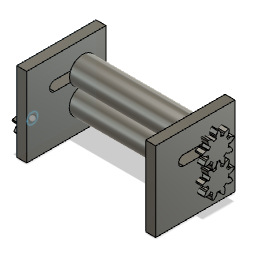
basic_parts (Autodesk Fusion 360 design; units mm, degrees)
Autodesk Fusion 360 part; units mm, degrees
sketch "biggear" plane through (0, 0, 0) normal (0, 1, 0) x (1, 0, 0)
  line L0 (141.1686, -145.633) -> (141.7294, -145.5695)
  line L1 (141.7294, -145.5695) -> (146.4127, -146.5108)
  line L2 (146.4127, -146.5108) -> (151.6977, -149.2435)
  line L3 (151.6977, -149.2435) -> (151.6977, -151.8334)
  line L4 (151.6977, -151.8334) -> (146.4127, -154.5661)
  line L5 (146.4127, -154.5661) -> (141.7294, -155.5074)
  line L6 (141.7294, -155.5074) -> (141.1687, -155.444)
  line L7 (141.1687, -155.444) -> (140.412, -159.9786)
  line L8 (140.412, -159.9786) -> (140.963, -160.1006)
  line L9 (140.963, -160.1006) -> (145.0868, -162.5116)
  line L10 (145.0868, -162.5116) -> (149.1982, -166.8123)
  line L11 (149.1982, -166.8123) -> (148.3573, -169.2618)
  line L12 (148.3573, -169.2618) -> (142.4713, -170.1304)
  line L13 (142.4713, -170.1304) -> (137.7361, -169.5001)
  line L14 (137.7361, -169.5001) -> (137.2263, -169.258)
  line L15 (137.2263, -169.258) -> (135.0383, -173.3012)
  line L16 (135.0383, -173.3012) -> (135.5198, -173.5955)
  line L17 (135.5198, -173.5955) -> (138.6373, -177.2149)
  line L18 (138.6373, -177.2149) -> (141.1295, -182.6175)
  line L19 (141.1295, -182.6175) -> (139.5388, -184.6613)
  line L20 (139.5388, -184.6613) -> (133.6897, -183.5717)
  line L21 (133.6897, -183.5717) -> (129.4158, -181.4379)
  line L22 (129.4158, -181.4379) -> (129.0122, -181.0435)
  line L23 (129.0122, -181.0435) -> (125.6299, -184.1571)
  line L24 (125.6299, -184.1571) -> (125.9897, -184.5919)
  line L25 (125.9897, -184.5919) -> (127.7632, -189.0274)
  line L26 (127.7632, -189.0274) -> (128.3661, -194.9465)
  line L27 (128.3661, -194.9465) -> (126.1979, -196.363)
  line L28 (126.1979, -196.363) -> (121.0195, -193.4332)
  line L29 (121.0195, -193.4332) -> (117.67, -190.0274)
  line L30 (117.67, -190.0274) -> (117.4164, -189.5232)
  line L31 (117.4164, -189.5232) -> (113.2064, -191.3699)
  line L32 (113.2064, -191.3699) -> (113.4055, -191.898)
  line L33 (113.4055, -191.898) -> (113.6427, -196.669)
  line L34 (113.6427, -196.669) -> (112.291, -202.4632)
  line L35 (112.291, -202.4632) -> (109.7804, -203.0989)
  line L36 (109.7804, -203.0989) -> (105.8339, -198.6465)
  line L37 (105.8339, -198.6465) -> (103.7717, -194.3376)
  line L38 (103.7717, -194.3376) -> (103.6955, -193.7784)
  line L39 (103.6955, -193.7784) -> (99.114, -194.158)
  line L40 (99.114, -194.158) -> (99.1309, -194.7221)
  line L41 (99.1309, -194.7221) -> (97.8061, -199.3117)
  line L42 (97.8061, -199.3117) -> (94.6462, -204.353)
  line L43 (94.6462, -204.353) -> (92.0652, -204.1391)
  line L44 (92.0652, -204.1391) -> (89.7783, -198.6465)
  line L45 (89.7783, -198.6465) -> (89.2269, -193.9015)
  line L46 (89.2269, -193.9015) -> (89.3365, -193.3478)
  line L47 (89.3365, -193.3478) -> (84.8799, -192.2193)
  line L48 (84.8799, -192.2193) -> (84.7127, -192.7583)
  line L49 (84.7127, -192.7583) -> (81.9694, -196.669)
  line L50 (81.9694, -196.669) -> (77.3439, -200.4112)
  line L51 (77.3439, -200.4112) -> (74.9722, -199.3708)
  line L52 (74.9722, -199.3708) -> (74.5926, -193.4332)
  line L53 (74.5926, -193.4332) -> (75.6118, -188.7663)
  line L54 (75.6118, -188.7663) -> (75.8952, -188.2782)
  line L55 (75.8952, -188.2782) -> (72.0465, -185.7638)
  line L56 (72.0465, -185.7638) -> (71.7134, -186.2193)
  line L57 (71.7134, -186.2193) -> (67.8489, -189.0274)
  line L58 (67.8489, -189.0274) -> (62.2589, -191.0649)
  line L59 (62.2589, -191.0649) -> (60.3535, -189.3108)
  line L60 (60.3535, -189.3108) -> (61.9225, -183.5716)
  line L61 (61.9225, -183.5716) -> (64.4018, -179.4885)
  line L62 (64.4018, -179.4885) -> (64.8283, -179.1189)
  line L63 (64.8283, -179.1189) -> (62.0046, -175.491)
  line L64 (62.0046, -175.491) -> (61.5416, -175.8137)
  line L65 (61.5416, -175.8137) -> (56.9748, -177.2149)
  line L66 (56.9748, -177.2149) -> (51.0261, -177.3269)
  line L67 (51.0261, -177.3269) -> (49.7935, -175.0492)
  line L68 (49.7935, -175.0492) -> (53.1409, -170.1304)
  line L69 (53.1409, -170.1304) -> (56.8117, -167.0736)
  line L70 (56.8117, -167.0736) -> (57.335, -166.8625)
  line L71 (57.335, -166.8625) -> (55.8423, -162.5143)
  line L72 (55.8423, -162.5143) -> (55.2996, -162.6692)
  line L73 (55.2996, -162.6692) -> (50.5253, -162.5116)
  line L74 (50.5253, -162.5116) -> (44.8626, -160.686)
  line L75 (44.8626, -160.686) -> (44.4363, -158.1315)
  line L76 (44.4363, -158.1315) -> (49.1995, -154.5661)
  line L77 (49.1995, -154.5661) -> (53.6639, -152.8668)
  line L78 (53.6639, -152.8668) -> (54.2275, -152.8371)
  line L79 (54.2275, -152.8371) -> (54.2275, -148.2398)
  line L80 (54.2275, -148.2398) -> (53.6639, -148.2101)
  line L81 (53.6639, -148.2101) -> (49.1995, -146.5108)
  line L82 (49.1995, -146.5108) -> (44.4363, -142.9454)
  line L83 (44.4363, -142.9454) -> (44.8626, -140.3909)
  line L84 (44.8626, -140.3909) -> (50.5253, -138.5654)
  line L85 (50.5253, -138.5654) -> (55.2996, -138.4077)
  line L86 (55.2996, -138.4077) -> (55.8423, -138.5626)
  line L87 (55.8423, -138.5626) -> (57.335, -134.2144)
  line L88 (57.335, -134.2144) -> (56.8117, -134.0033)
  line L89 (56.8117, -134.0033) -> (53.1409, -130.9465)
  line L90 (53.1409, -130.9465) -> (49.7934, -126.0277)
  line L91 (49.7934, -126.0277) -> (51.0261, -123.75)
  line L92 (51.0261, -123.75) -> (56.9748, -123.8621)
  line L93 (56.9748, -123.8621) -> (61.5416, -125.2632)
  line L94 (61.5416, -125.2632) -> (62.0046, -125.5859)
  line L95 (62.0046, -125.5859) -> (64.8283, -121.958)
  line L96 (64.8283, -121.958) -> (64.4018, -121.5884)
  line L97 (64.4018, -121.5884) -> (61.9225, -117.5053)
  line L98 (61.9225, -117.5053) -> (60.3535, -111.7661)
  line L99 (60.3535, -111.7661) -> (62.2589, -110.0121)
  line L100 (62.2589, -110.0121) -> (67.8489, -112.0496)
  line L101 (67.8489, -112.0496) -> (71.7134, -114.8576)
  line L102 (71.7134, -114.8576) -> (72.0465, -115.3132)
  line L103 (72.0465, -115.3132) -> (75.8952, -112.7987)
  line L104 (75.8952, -112.7987) -> (75.6118, -112.3106)
  line L105 (75.6118, -112.3106) -> (74.5926, -107.6437)
  line L106 (74.5926, -107.6437) -> (74.9722, -101.7061)
  line L107 (74.9722, -101.7061) -> (77.3439, -100.6657)
  line L108 (77.3439, -100.6657) -> (81.9694, -104.4079)
  line L109 (81.9694, -104.4079) -> (84.7127, -108.3186)
  line L110 (84.7127, -108.3186) -> (84.8799, -108.8576)
  line L111 (84.8799, -108.8576) -> (89.3364, -107.7291)
  line L112 (89.3364, -107.7291) -> (89.2269, -107.1755)
  line L113 (89.2269, -107.1755) -> (89.7783, -102.4305)
  line L114 (89.7783, -102.4305) -> (92.0652, -96.9378)
  line L115 (92.0652, -96.9378) -> (94.6462, -96.7239)
  line L116 (94.6462, -96.7239) -> (97.8061, -101.7653)
  line L117 (97.8061, -101.7653) -> (99.1309, -106.3548)
  line L118 (99.1309, -106.3548) -> (99.114, -106.9189)
  line L119 (99.114, -106.9189) -> (103.6955, -107.2985)
  line L120 (103.6955, -107.2985) -> (103.7717, -106.7393)
  line L121 (103.7717, -106.7393) -> (105.8339, -102.4305)
  line L122 (105.8339, -102.4305) -> (109.7804, -97.978)
  line L123 (109.7804, -97.978) -> (112.291, -98.6138)
  line L124 (112.291, -98.6138) -> (113.6427, -104.4079)
  line L125 (113.6427, -104.4079) -> (113.4055, -109.179)
  line L126 (113.4055, -109.179) -> (113.2064, -109.707)
  line L127 (113.2064, -109.707) -> (117.4164, -111.5537)
  line L128 (117.4164, -111.5537) -> (117.67, -111.0495)
  line L129 (117.67, -111.0495) -> (121.0195, -107.6437)
  line L130 (121.0195, -107.6437) -> (126.1979, -104.7139)
  line L131 (126.1979, -104.7139) -> (128.3661, -106.1304)
  line L132 (128.3661, -106.1304) -> (127.7632, -112.0496)
  line L133 (127.7632, -112.0496) -> (125.9897, -116.4851)
  line L134 (125.9897, -116.4851) -> (125.6299, -116.9198)
  line L135 (125.6299, -116.9198) -> (129.0122, -120.0335)
  line L136 (129.0122, -120.0335) -> (129.4158, -119.639)
  line L137 (129.4158, -119.639) -> (133.6897, -117.5053)
  line L138 (133.6897, -117.5053) -> (139.5388, -116.4156)
  line L139 (139.5388, -116.4156) -> (141.1295, -118.4594)
  line L140 (141.1295, -118.4594) -> (138.6373, -123.8621)
  line L141 (138.6373, -123.8621) -> (135.5198, -127.4814)
  line L142 (135.5198, -127.4814) -> (135.0383, -127.7757)
  line L143 (135.0383, -127.7757) -> (137.2263, -131.8189)
  line L144 (137.2263, -131.8189) -> (137.7361, -131.5768)
  line L145 (137.7361, -131.5768) -> (142.4713, -130.9465)
  line L146 (142.4713, -130.9465) -> (148.3573, -131.8151)
  line L147 (148.3573, -131.8151) -> (149.1982, -134.2646)
  line L148 (149.1982, -134.2646) -> (145.0868, -138.5653)
  line L149 (145.0868, -138.5653) -> (140.9629, -140.9763)
  line L150 (140.9629, -140.9763) -> (140.412, -141.0984)
  line L151 (140.412, -141.0984) -> (141.1686, -145.633)
sketch "smallgear" plane through (0, 0, 0) normal (0, 1, 0) x (-1, 0, 0)
  line L0 (42.6523, 16.1607) -> (47.1357, 13.5722)
  line L1 (64.2228, -1.5259) -> (58.7553, -4.5447)
  line L2 (43.751, 18.9194) -> (42.6523, 16.1607)
  line L3 (21.0334, -24.4753) -> (21.1528, -18.2309)
  line L4 (53.5978, -4.1821) -> (51.8271, -9.047)
  line L5 (54.4421, 9.3882) -> (51.8271, 7.9812)
  line L6 (56.9824, -19.4328) -> (50.8535, -18.2309)
  line L7 (58.2589, 16.8457) -> (56.011, 11.0187)
  line L8 (41.8813, -28.1514) -> (39.9256, -28.4962)
  line L9 (28.1014, 21.1769) -> (29.4347, 19.3487)
  line L10 (13.2511, 3.4789) -> (9.1458, 8.1857)
  line L11 (15.9953, -12.0844) -> (9.825, -11.1177)
  line L12 (22.7533, 24.4025) -> (28.1014, 21.1769)
  line L13 (21.1528, 17.1651) -> (21.0334, 23.4096)
  line L14 (56.011, 11.0187) -> (54.4421, 9.3882)
  line L15 (51.8271, 7.9812) -> (53.5978, 3.1164)
  line L16 (50.8535, 17.1651) -> (56.9824, 18.367)
  line L17 (35.4646, -18.4939) -> (30.3662, -17.5949)
  line L18 (48.9754, 15.9031) -> (50.8535, 17.1651)
  line L19 (22.7533, -25.4683) -> (21.0334, -24.4753)
  line L20 (41.8813, 27.0856) -> (43.9049, 21.1769)
  line L21 (58.7553, -4.5447) -> (56.5053, -4.7852)
  line L22 (56.5053, 3.7194) -> (58.7553, 3.4789)
  line L23 (9.1458, -9.2515) -> (13.2511, -4.5447)
  line L24 (51.8271, -9.047) -> (54.4421, -10.454)
  line L25 (9.1458, 8.1857) -> (9.825, 10.0519)
  line L26 (21.0334, 23.4096) -> (22.7533, 24.4025)
  line L27 (36.0032, 22.5702) -> (39.9256, 27.4305)
  line L28 (18.2215, 2.0556) -> (15.283, 2.4834)
  line L29 (9.825, 10.0519) -> (15.9953, 11.0187)
  line L30 (18.2215, -3.1214) -> (18.2215, 2.0556)
  line L31 (35.4646, 17.4281) -> (35.3756, 20.3962)
  line L32 (15.283, -3.5492) -> (18.2215, -3.1214)
  line L33 (13.2511, -4.5447) -> (15.283, -3.5492)
  line L34 (29.4347, 19.3487) -> (30.3662, 16.5291)
  line L35 (30.3662, 16.5291) -> (35.4646, 17.4281)
  line L36 (28.1014, -22.2427) -> (22.7533, -25.4683)
  line L37 (30.3662, -17.5949) -> (29.4347, -20.4144)
  line L38 (35.3756, -21.462) -> (35.4646, -18.4939)
  line L39 (43.9049, -22.2427) -> (41.8813, -28.1514)
  line L40 (39.9256, 27.4305) -> (41.8813, 27.0856)
  line L41 (56.011, -12.0844) -> (58.2589, -17.9115)
  line L42 (54.4421, -10.454) -> (56.011, -12.0844)
  line L43 (36.0032, -23.636) -> (35.3756, -21.462)
  line L44 (43.751, -19.9852) -> (43.9049, -22.2427)
  line L45 (56.5053, -4.7852) -> (53.5978, -4.1821)
  line L46 (47.1357, -14.638) -> (42.6523, -17.2265)
  line L47 (22.0695, 15.0964) -> (21.1528, 17.1651)
  line L48 (20.7178, 8.914) -> (24.0455, 12.8799)
  line L49 (15.283, 2.4834) -> (13.2511, 3.4789)
  line L50 (35.3756, 20.3962) -> (36.0032, 22.5702)
  line L51 (47.1357, 13.5722) -> (48.9754, 15.9031)
  line L52 (50.8535, -18.2309) -> (48.9754, -16.9689)
  line L53 (18.1918, -11.5409) -> (15.9953, -12.0844)
  line L54 (58.2589, -17.9115) -> (56.9824, -19.4328)
  line L55 (43.9049, 21.1769) -> (43.751, 18.9194)
  line L56 (22.0695, -16.1621) -> (24.0455, -13.9456)
  line L57 (9.825, -11.1177) -> (9.1458, -9.2515)
  line L58 (42.6523, -17.2265) -> (43.751, -19.9852)
  line L59 (64.2228, 0.4601) -> (64.2228, -1.5259)
  line L60 (39.9256, -28.4962) -> (36.0032, -23.636)
  line L61 (20.7178, -9.9798) -> (18.1918, -11.5409)
  line L62 (56.9824, 18.367) -> (58.2589, 16.8457)
  line L63 (58.7553, 3.4789) -> (64.2228, 0.4601)
  line L64 (29.4347, -20.4144) -> (28.1014, -22.2427)
  line L65 (24.0455, -13.9456) -> (20.7178, -9.9798)
  line L66 (15.9953, 11.0187) -> (18.1918, 10.4751)
  line L67 (24.0455, 12.8799) -> (22.0695, 15.0964)
  line L68 (48.9754, -16.9689) -> (47.1357, -14.638)
  line L69 (21.1528, -18.2309) -> (22.0695, -16.1621)
  line L70 (18.1918, 10.4751) -> (20.7178, 8.914)
  line L71 (53.5978, 3.1164) -> (56.5053, 3.7194)
scale "Scale1" [no effect]
scale "Scale2" [no effect]
extrude "Extrude3" add sketch "biggear" along normal blind 12.7 makes body 1
extrude "Extrude4" add sketch "smallgear" along normal blind 12.7 separate body makes body 2
cylinder "CylinderPrimitive1" add diameter 50.8 height 228.6 placed x (1, 0, 0) y (0, 0, -1) z (0, 1, 0) at (-75, 0, 125) separate body makes body 3
cylinder "CylinderPrimitive2" cut diameter 38.1 height 228.6 placed x (1, 0, 0) y (0, 0, -1) z (0, 1, 0) at (-75, 0, 125) bodies 3
cylinder "CylinderPrimitive3" add diameter 38.1 height 19.55 placed x (1, 0, 0) y (0, 0, -1) z (0, 1, 0) at (20, 0, 60) separate body makes body 4
cylinder "CylinderPrimitive4" cut diameter 25.4 height 19.55 placed x (1, 0, 0) y (0, 0, -1) z (0, 1, 0) at (20, 0, 60) bodies 4
sketch "Sketch9" plane through (0, 0, 0) normal (0, 1, 0) x (1, 0, 0)
box "BoxPrimitive1" add length 152.4 width 19.05 height 152.4 placed x (0, 0, -1) y (-1, 0, 0) z (0, 1, 0) at (19.05, 0, 0) separate body makes body 5
copy_body "CopyPasteBodies1" bodies 5 makes body 6
move_body "Move1" bodies 6 to x (1, 0, 0) y (0, 1, 0) z (0, 0, 1) at (247.65, 0, 0)
copy_body "CopyPasteBodies2" bodies 3 makes body 7
move_body "Move2" bodies 7 to x (1, 0, 0) y (0, 1, 0) z (0, 0, 1) at (-125, 0, 0)
copy_body "Body->Comp1" bodies 1 removing the originals makes body 8 in component "Component"
copy_body "Body->Comp2" bodies 2 removing the originals makes body 9 in component "Component'"
copy_body "Body->Comp3" bodies 3 removing the originals makes body 10 in component "Component''"
copy_body "Body->Comp4" bodies 4 removing the originals makes body 11 in component "Component'''"
copy_body "Body->Comp6" bodies 6 removing the originals makes body 12 in component "Component''''"
copy_body "Body->Comp7" bodies 7 removing the originals makes body 13 in component "Component'''''"
sketch "Sketch10" plane through (266.7, 0, 0) normal (1, 0, 0) x (0, 0, -1)
  line L0 (0, 152.4) -> (0, 0)
  line L1 (0, 0) -> (152.4, 0)
  line L2 (152.4, 0) -> (152.4, 152.4)
  line L3 (152.4, 152.4) -> (0, 152.4)
  line L4 (0, 76.2) -> (152.4, 76.2) construction
  line L5 (0, 76.2) -> (0, 101.6) construction
  line L6 (152.4, 76.2) -> (152.4, 50.8) construction
  line L7 (0, 101.6) -> (152.4, 101.6) construction
  line L8 (152.4, 50.8) -> (0, 50.8) construction
  dimension "d31" = 25.4
  dimension "d32" = 25.4
  constraint midpoint L0 L4.start
  constraint midpoint L2 L4.end
  constraint perpendicular L4 L5
  constraint perpendicular L4 L6
  constraint coincident L2 L7.end
  constraint perpendicular L2 L7
  constraint coincident L0 L8.end
  constraint perpendicular L0 L8
  measures "d31" distance of L4.start L5.end
  measures "d32" distance of L4.end L6.end
cylinder "CylinderPrimitive1'" cut diameter 38.1 height -35 placed x (0, 0, -1) y (0, 1, 0) z (1, 0, 0) at (266.7, 50.846, -107.6952) bodies 12 in component "Component''''"
cylinder "CylinderPrimitive2'" cut diameter 19.05 height -70 placed x (0, 0, -1) y (0, 1, 0) z (1, 0, 0) at (266.7, 101.6458, -53.5935) bodies 12 in component "Component''''"
cylinder "CylinderPrimitive3'" cut diameter 19.05 height -60 placed x (0, 0, -1) y (0, 1, 0) z (1, 0, 0) at (266.7, 101.5399, -107.6629) bodies 12 in component "Component''''"
box "BoxPrimitive1'" cut length 19.1715 width 54.945 height -95 placed x (0, 1, 0) y (0, 0, 1) z (1, 0, 0) at (266.7, 92.053, -108.4535) bodies 12 in component "Component''''"
cylinder "CylinderPrimitive5" add diameter 38.1 height 19.05 placed x (1, 0, 0) y (0, 0, -1) z (0, 1, 0) at (80, 0, 70) separate body makes body 14
cylinder "CylinderPrimitive6" add diameter 19.05 height -19.05 placed x (1, 0, 0) y (0, 0, -1) z (0, 1, 0) at (80, 0, 70) bodies 14
copy_body "CopyPasteBodies3" bodies 14 makes body 15
copy_body "Body->Comp8" bodies 15 removing the originals makes body 16 in component "Component''''''"
copy_body "Body->Comp9" bodies 14 removing the originals makes body 17 in component "Component'''''''"
sketch "Sketch17" plane through (0, 0, 0) normal (-1, 0, 0) x (0, 0, 1)
  line L0 (-53.5085, 92.053) -> (-106.8119, 92.053)
  arc A0 (-108.4535, 111.032) -> (-106.8119, 92.053) centre (-107.6629, 101.5399) ccw
  line L1 (-108.4535, 111.032) -> (-108.4535, 111.2245)
  line L2 (-108.4535, 111.2245) -> (-53.5085, 111.2245)
  line L3 (-53.5085, 111.2245) -> (-53.5085, 111.1704)
  arc A1 (-53.5085, 92.1211) -> (-53.5085, 111.1704) centre (-53.5935, 101.6458) ccw
  line L4 (-53.5085, 92.1211) -> (-53.5085, 92.053)
  circle A2 centre (-107.6952, 50.846) radius 19.05
  line L5 (-152.4, 152.4) -> (-152.4, 0)
  line L6 (-152.4, 0) -> (0, 0)
  line L7 (0, 0) -> (0, 152.4)
  line L8 (0, 152.4) -> (-152.4, 152.4)
  circle A3 centre (-30, 50) radius 10
scale "Scale1'" factor 1.1 about (-53.5978, 0, -4.1821) bodies 9 in component "Component'"
component "Component" placed x (0, -1, 0) y (1, 0, 0) z (0, 0, 1) at (-13.7, 148.913, -258.2337)
component "Component'" placed x (0, -1, 0) y (1, 0, 0) z (0, 0, 1) at (-12.7, 13.3157, -34.4671)
component "Component''" placed x (0, -1, 0) y (1, 0, 0) z (0, 0, 1) at (19.05, 26.5399, -232.6629)
component "Component'''" placed x (0, -1, 0) y (-1, 0, 0) z (0, 0, -1) at (266.7, 70.846, -47.6952)
component "Component''''" placed x (1, 0, 0) y (0, 1, 0) z (0, 0, 1) at (0, 0, 0)
component "Component'''''" placed x (0, -1, 0) y (1, 0, 0) z (0, 0, 1) at (18.55, -149.154, -232.6952)
component "Component''''" placed x (1, 0, 0) y (0, 1, 0) z (0, 0, 1) at (-247.65, 0, 0)
component "Component'''" placed x (0, -1, 0) y (1, 0, 0) z (0, 0, 1) at (-1, 70.846, -167.6952)
component "Component''''''" placed x (0, -1, 0) y (1, 0, 0) z (0, 0, 1) at (19.05, 181.5399, -177.6629)
component "Component'''''''" placed x (0, -1, 0) y (-1, 0, 0) z (0, 0, -1) at (247.65, 181.5399, -37.6629)
component "Component'" placed x (0, -1, 0) y (-1, 0, 0) z (0, 0, -1) at (279.4, 64.8556, -108.1958)
component "Component'" placed x (0, -1, 0) y (-1, 0, 0) z (0, 0, -1) at (279.4, 14.1617, -108.2281)
hidden bodies 5
equation "projwidth = 9 in"
equation "gearthickness = ( 1 / 2 ) * 1 in"
equation "rollerwidth = 2 in"
equation "rollerthickness = ( 1 / 4 ) * 1 in"
equation "d11 = gearthickness"
equation "d13 = gearthickness"
equation "d15 = projwidth"
equation "d17 = projwidth"
equation "woodthickness = ( 3 / 4 ) * 1 in"
equation "d20 = woodthickness + 0.5 mm"
equation "d22 = woodthickness + 0.5 mm"
equation "projlength = 6 in"
equation "projheight = 6 in"
equation "d28 = projheight"
equation "d31 = rollerwidth / 2"
equation "d32 = rollerwidth / 2"
equation "smallroler = 0.75 in"
equation "d81 = woodthickness"
equation "d83 = -woodthickness"
